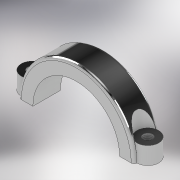
# Autodesk Inventor part: Pistonhandattacher
Saved by Autodesk Inventor 2019 (Build 230136000, 136)
## iProperties
Created: 2020-05-28
Part Number: Pistonhandattacher
Material: Generic
Document SubType Name: Modeling
Designer: Manoj
Density: 1 g/cm^3
Appearance: Chrome - Polished
Author: Manoj
Autodesk Inventor part; units mm, degrees
ref_plane "YZ Plane" through (0, 0, 0) normal (1, 0, 0) x (0, 1, 0)
ref_plane "XZ Plane" through (0, 0, 0) normal (0, 1, 0) x (-1, 0, 0)
ref_plane "XY Plane" through (0, 0, 0) normal (0, 0, 1) x (1, 0, 0)
sketch "Sketch1" plane through (0, 0, 0) normal (0, 0, 1) x (1, 0, 0)
  arc A0 (38.1, 0) -> (-38.1, 0) centre (0, 0) ccw
  arc A1 (50.8, 0) -> (-50.8, 0) centre (0, 0) ccw
  line L0 (-50.8, 0) -> (-38.1, 0)
  line L1 (38.1, 0) -> (50.8, 0)
  dimension "d0" = 76.2
  dimension "d1" = 12.7
  constraints: 4 end point, 4 point on circle, 2 centre point, 2 point on line, 1 coincident, 1 horizontal, 1 horizontal alignment
  measures "d0" diameter of A0
  measures "d1" radial gap between concentric circles of A0 A1
extrude "Extrusion1" add sketch "Sketch1" along normal blind 24.13
sketch "Sketch2" plane through (38.1, 0, 0) normal (0, -1, 0) x (1, 0, 0)
  line L0 (12.7, 0) -> (12.7, 24.13) construction
  circle A0 centre (12.7, 12.065) radius 9.525
  point P0 (-38.1, 0)
  dimension "d4" = 19.05
  constraints: 1 centre point, 1 midpoint
  measures "d4" diameter of A0
extrude "Extrusion2" add sketch "Sketch2" against normal blind 15.25
sketch "Sketch3" plane through (38.1, 15.25, 0) normal (0, 1, 0) x (1, 0, 0)
  arc A0 (12.7, -21.59) -> (12.7, -2.54) centre (12.7, -12.065) ccw projected
  circle A1 centre (12.7, -12.065) radius 9.525
  point P0 (-38.1, 0)
  dimension "d7" = 19.05
  constraints: 1 centre point, 1 coincident
  measures "d7" diameter of A1
extrude "Extrusion3" cut sketch "Sketch3" along normal blind 15.25 draft 3
sketch "Sketch4" plane through (38.1, 15.25, 0) normal (0, 1, 0) x (1, 0, 0)
  arc A0 (10.357, -21.2973) -> (10.357, -2.8327) centre (12.7, -12.065) ccw projected
  point P0 (-38.1, 0)
  constraints: 1 coincident
hole "Hole1" at (50.8, 15.25, 12.065) direction (0, -1, 0) diameter 8.433 end through all clearance for "Socket Head Cap Screw" size "5/16" standard "Ansi Unified Screw Threads"
mirror "Mirror1" about plane through (0, 0, 0) normal (1, 0, 0) of "Extrusion2", "Extrusion3", "Hole1"
fillet "Fillet1" radius 2.54 2 edges at (0, 50.8, 24.13) (0, 50.8, 0)
thread "Thread1" size "M9x1.25" class "6H" standard "ANSI Metric M Profile" full length
thread "Thread2" size "M9x1.25" class "6H" standard "ANSI Metric M Profile" full length
body "Solid1"
